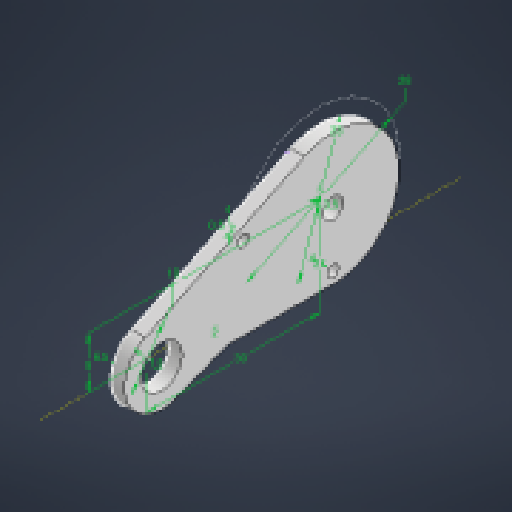
# Autodesk Inventor part: Gear_Cover
Saved by Autodesk Inventor 2024.2 (Build 282272000, 272)
## iProperties
Created: 2024-02-26
Part Number: Gear_Cover
Material: 一般
Document SubType Name: Modeling
Designer: Hanaoka
Density: 1 g/cm^3
Appearance: 既定
Author: Hanaoka
Autodesk Inventor part; units mm, degrees
ref_plane "YZ Plane" through (0, 0, 0) normal (1, 0, 0) x (0, 1, 0)
ref_plane "XZ Plane" through (0, 0, 0) normal (0, 1, 0) x (-1, 0, 0)
ref_plane "XY Plane" through (0, 0, 0) normal (0, 0, 1) x (1, 0, 0)
sketch "スケッチ1" plane through (0, 0, 0) normal (1, 0, 0) x (0, 1, 0)
  circle A0 centre (0, 0) radius 3.6
  arc A1 (5.8479, 2.8377) -> (-6.0569, -2.3587) centre (0, 0) ccw
  line L0 (-6.0569, -2.3587) -> (-2.6363, -11.1423)
  line L1 (-2.5, -11.8681) -> (-2.5, -30)
  line L2 (0, -54.5111) -> (0, 19.0665) construction
  circle A2 centre (0, 0) radius 5 construction
  line L3 (4.8885, 1.0499) -> (11.4443, -29.4751) construction
  line L4 (-4.6592, -1.8144) -> (6.6704, -30.9072) construction
  circle A3 centre (9, -30) radius 14 construction
  circle A4 centre (9, -30) radius 2.5 construction
  circle A5 centre (9, -30) radius 11.5
  arc A6 (-2.5, -11.8681) -> (-2.6363, -11.1423) centre (-4.5, -11.8681) ccw
  line L5 (5.8479, 2.8377) -> (19.3462, -24.9795)
  circle A7 centre (9, -30) radius 1.75
  circle A8 centre (11.9263, -14.2699) radius 2
  circle A9 centre (11.9263, -14.2699) radius 1
  arc A10 (12.3074, -12.3065) -> (12.8525, -11.5974) centre (12.4027, -11.8157) ccw
  arc A11 (14.5988, -15.1961) -> (13.7044, -15.1855) centre (14.149, -15.4144) ccw
  circle A12 centre (-0.5, -30) radius 1
  circle A13 centre (-0.5, -30) radius 2
  line L6 (9, -30) -> (-2.5, -30)
  point P0 (-2.5, -11.4924)
  point P1 (19.0229, -24.3617)
  point P2 (13.7257, -13.3967)
  dimension "d0" = 7.2
  dimension "d1" = 6.5
  dimension "d3" = 10
  dimension "d4" = 28
  dimension "d5" = 5
  dimension "d6" = 23
  dimension "d10" = 30
  dimension "d11" = 9
  dimension "d12" = 3.5
  dimension "d13" = 2
  dimension "d14" = 2
  dimension "d15" = 4
  dimension "d18" = 0.5
  dimension "d19" = 2
  dimension "d20" = 4
  constraints: 17 point on circle, 17 tangent, 14 centre point, 12 end point, 8 coincident, 5 point on line, 1 equal radius, 1 horizontal, 1 parallel, 1 vertical
  measures "d0" diameter of A0
  measures "d1" radius of A1
  measures "d3" diameter of A2
  measures "d4" diameter of A3
  measures "d5" diameter of A4
  measures "d6" diameter of A5
  measures "d10" vertical distance of A3.centre point (0, 0)
  measures "d11" horizontal distance of A3.centre point (0, 0)
  measures "d12" diameter of A7
  measures "d13" radius of A6
  measures "d14" diameter of A9
  measures "d15" diameter of A8
  measures "d18" radius of A10
  measures "d19" diameter of A12
  measures "d20" diameter of A13
extrude "押し出し1" add sketch "スケッチ1" along normal blind 2.5 contours L5 A10 A8 A11 A5 L1 A6 L0 A1 | L5 A8 A10 | L5 A11 A8 | A8 | A5 | L6 A12 A13 | A13 L6 A12
